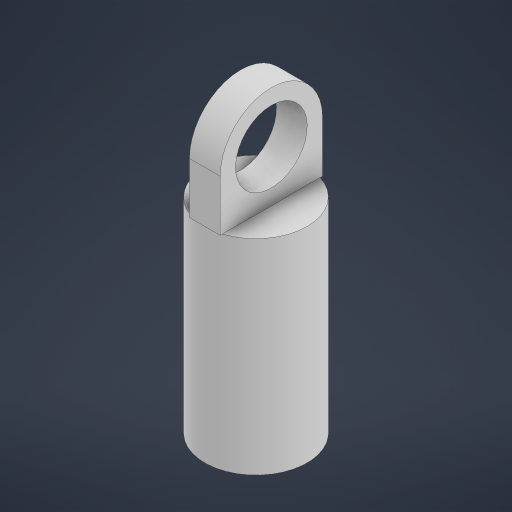
# Autodesk Inventor part: FP V2 Z Axis connector
Saved by Autodesk Inventor 2023.6 (Build 276521000, 521)
## iProperties
Created: 2026-02-25
Part Number: FP V2 Z Axis connector
Material: Generic
Document SubType Name: Modeling
Designer: user
Density: 1 g/cm^3
Appearance: Default
Author: user
Autodesk Inventor part; units mm, degrees
ref_plane "YZ Plane" through (0, 0, 0) normal (1, 0, 0) x (0, 1, 0)
ref_plane "XZ Plane" through (0, 0, 0) normal (0, 1, 0) x (-1, 0, 0)
ref_plane "XY Plane" through (0, 0, 0) normal (0, 0, 1) x (1, 0, 0)
sketch "Sketch3" plane through (0, 0, 0) normal (0, 1, 0) x (-1, 0, 0)
  circle A0 centre (0, 0) radius 5
  dimension "d8" = 10
  constraints: 1 centre point, 1 coincident
  measures "d8" diameter of A0
extrude "Extrusion3" add sketch "Sketch3" along normal blind 20
sketch "Sketch4" plane through (0, 0, 0) normal (1, 0, 0) x (0, 1, 0)
  circle A0 centre (25, 0) radius 3.5
  circle A1 centre (25, 0) radius 5
  line L0 (20, -5) -> (20, 5) projected
  line L1 (20, -5) -> (25, -5)
  line L2 (20, 5) -> (25, 5)
  point P0 (0, 0)
  point P1 (25, 5)
  point P2 (52.9865, 4.5767)
  point P3 (20, 0)
  dimension "d11" = 7
  dimension "d12" = 10
  constraints: 4 end point, 3 point on circle, 3 tangent, 2 centre point, 1 coincident
  measures "d11" diameter of A0
  measures "d12" diameter of A1
extrude "Extrusion4" add sketch "Sketch4" along normal mid plane 3
body "Solid2"
